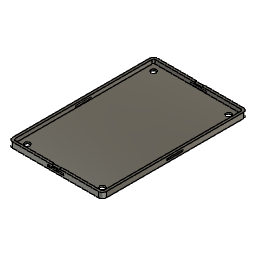
Backcover+small (Autodesk Fusion 360 design; units mm, degrees)
Autodesk Fusion 360 part; units mm, degrees
sketch "Sketch1" plane through (0, 0, 0) normal (0, 0, 1) x (1, 0, 0)
  circle A0 centre (14.5, 177.5) radius 3.5
  line L0 (7.5, 189.5) -> (118.5, 189.5)
  line L1 (123.5, 184.5) -> (123.5, 7.5)
  line L2 (118.5, 2.5) -> (7.5, 2.5)
  line L3 (2.5, 7.5) -> (2.5, 184.5)
  arc A1 (7.5, 189.5) -> (2.5, 184.5) centre (7.5, 184.5) ccw
  arc A2 (123.5, 184.5) -> (118.5, 189.5) centre (118.5, 184.5) ccw
  arc A3 (2.5, 7.5) -> (7.5, 2.5) centre (7.5, 7.5) ccw
  arc A4 (118.5, 2.5) -> (123.5, 7.5) centre (118.5, 7.5) ccw
  arc A5 (118.5, 5.5) -> (120.5, 7.5) centre (118.5, 7.5) ccw
  line L4 (120.5, 184.5) -> (120.5, 7.5)
  arc A6 (120.5, 184.5) -> (118.5, 186.5) centre (118.5, 184.5) ccw
  line L5 (7.5, 186.5) -> (118.5, 186.5)
  arc A7 (7.5, 186.5) -> (5.5, 184.5) centre (7.5, 184.5) ccw
  line L6 (5.5, 7.5) -> (5.5, 184.5)
  arc A8 (5.5, 7.5) -> (7.5, 5.5) centre (7.5, 7.5) ccw
  line L7 (118.5, 5.5) -> (7.5, 5.5)
  line L8 (63, 186.5) -> (63, 5.5)
  line L9 (5.5, 96) -> (120.5, 96)
  circle A9 centre (111.5, 177.5) radius 3.5
  circle A10 centre (14.5, 14.5) radius 3.5
  circle A11 centre (111.5, 14.5) radius 3.5
  dimension "d5" = 7
  dimension "d28" = 5
  dimension "d30" = 5
  dimension "d32" = 5
  dimension "d34" = 5
  dimension "d36" = 3
  dimension "d37" = 187
  dimension "d38" = 121
  dimension "d41" = 9
  dimension "d42" = 9
  constraint horizontal L0
  constraint perpendicular L0 L1
  constraint parallel L0 L2
  constraint parallel L1 L3
  constraint tangent L3 A1
  constraint tangent L0 A1
  constraint tangent L0 A2
  constraint tangent L1 A2
  constraint tangent L3 A3
  constraint tangent L2 A3
  constraint tangent L1 A4
  constraint tangent L2 A4
  constraint midpoint L5 L8.start
  constraint midpoint L7 L8.end
  constraint perpendicular L7 L8
  constraint midpoint L6 L9.start
  constraint midpoint L4 L9.end
  constraint perpendicular L4 L9
  constraint symmetric A0 L8 A9
  constraint symmetric A0 L9 A10
  constraint symmetric L9 A9 A11
  measures "d5" diameter of A0
  measures "d28" radius of A1
  measures "d30" radius of A2
  measures "d32" radius of A3
  measures "d34" radius of A4
  measures "d37" distance of L0 L2
  measures "d38" distance of L1 L3
  measures "d41" distance of A0.centre L5
  measures "d42" distance of A0.centre L6
extrude "Extrude5" add sketch "Sketch1" along normal blind 2 contours L0 L1 L2 L3 A1 A2 A3 A4 | A5 L4 L7 L8 L9 | L6 A8 L7 L8 L9 | L4 A6 L5 L8 L9 | L5 A7 L6 L8 L9
extrude "Extrude6" add sketch "Sketch1" along normal blind 7 contours L0 L1 L2 L3 A1 A2 A3 A4
sketch "Skizze3" plane through (2.5, 0, 0) normal (-1, 0, 0) x (0, -1, 0)
  line L0 (-184.5, 0) -> (-7.5, 0)
  line L1 (-7.5, 0) -> (-7.5, 7)
  line L2 (-7.5, 7) -> (-184.5, 7)
  line L3 (-184.5, 7) -> (-184.5, 0)
  line L4 (-184.5, 7) -> (-7.5, 0)
  line L5 (-7.5, 7) -> (-184.5, 0)
  line L6 (-85.75, 4.5) -> (-106.25, 4.5)
  line L7 (-106.25, 4.5) -> (-106.25, 2.5)
  line L8 (-106.25, 2.5) -> (-85.75, 2.5)
  line L9 (-85.75, 2.5) -> (-85.75, 4.5)
  line L10 (-85.75, 4.5) -> (-106.25, 2.5) construction
  line L11 (-106.25, 4.5) -> (-85.75, 2.5) construction
  point P0 (-96, 3.5)
  dimension "d43" = 20.5
  dimension "d44" = 2
  constraint coincident L2.end L3.start
  constraint coincident L0.end L1.start
  constraint coincident L1.end L2.start
  constraint coincident L0.start L3.end
  constraint horizontal L6
  constraint perpendicular L6 L7
  constraint parallel L6 L8
  constraint parallel L7 L9
  constraint coincident L10 P0
  constraint coincident L11 P0
  constraint midpoint L5 P0
  measures "d43" distance of L7.end L8.end
  measures "d44" distance of L6.end L7.end
extrude "Extrusion7" cut sketch "Skizze3" against normal blind 2.5 contours L4 L5 L7 | L4 L5 L7 L8 L9 | L4 L5 L9 | L4 L5 L6 L7 L9
sketch "Skizze4" plane through (0, 189.5, 0) normal (0, 1, 0) x (-1, 0, 0)
  line L0 (-118.5, 0) -> (-7.5, 0)
  line L1 (-7.5, 0) -> (-7.5, 7)
  line L2 (-7.5, 7) -> (-118.5, 7)
  line L3 (-118.5, 7) -> (-118.5, 0)
  line L4 (-118.5, 7) -> (-7.5, 0)
  line L5 (-7.5, 7) -> (-118.5, 0)
  line L6 (-52.75, 4.5) -> (-73.25, 4.5)
  line L7 (-73.25, 4.5) -> (-73.25, 2.5)
  line L8 (-73.25, 2.5) -> (-52.75, 2.5)
  line L9 (-52.75, 2.5) -> (-52.75, 4.5)
  line L10 (-52.75, 4.5) -> (-73.25, 2.5) construction
  line L11 (-73.25, 4.5) -> (-52.75, 2.5) construction
  point P0 (-63, 3.5)
  dimension "d47" = 20.5
  dimension "d48" = 2
  constraint coincident L2.end L3.start
  constraint coincident L0.end L1.start
  constraint coincident L1.end L2.start
  constraint coincident L0.start L3.end
  constraint horizontal L6
  constraint perpendicular L6 L7
  constraint parallel L6 L8
  constraint parallel L7 L9
  constraint coincident L10 P0
  constraint coincident L11 P0
  constraint midpoint L4 P0
  measures "d47" distance of L7.end L8.end
  measures "d48" distance of L6.end L7.end
extrude "Extrusion8" cut sketch "Skizze4" against normal blind 2.5 contours L4 L5 L7 | L4 L5 L7 L8 L9 | L4 L5 L9 | L4 L5 L6 L7 L9
sketch "Skizze5" plane through (0, 2.5, 0) normal (0, -1, 0) x (1, 0, 0)
  line L0 (7.5, 0) -> (118.5, 0)
  line L1 (118.5, 0) -> (118.5, 7)
  line L2 (118.5, 7) -> (7.5, 7)
  line L3 (7.5, 7) -> (7.5, 0)
  line L4 (118.5, 7) -> (7.5, 0)
  line L5 (7.5, 7) -> (118.5, 0)
  line L6 (73.25, 4.5) -> (52.75, 4.5)
  line L7 (52.75, 4.5) -> (52.75, 2.5)
  line L8 (52.75, 2.5) -> (73.25, 2.5)
  line L9 (73.25, 2.5) -> (73.25, 4.5)
  line L10 (73.25, 4.5) -> (52.75, 2.5) construction
  line L11 (52.75, 4.5) -> (73.25, 2.5) construction
  point P0 (63, 3.5)
  dimension "d51" = 20.5
  dimension "d52" = 2
  constraint coincident L1.end L2.start
  constraint coincident L0.start L3.end
  constraint coincident L2.end L3.start
  constraint coincident L0.end L1.start
  constraint horizontal L6
  constraint perpendicular L6 L7
  constraint parallel L6 L8
  constraint parallel L7 L9
  constraint coincident L10 P0
  constraint coincident L11 P0
  constraint midpoint L5 P0
  measures "d51" distance of L7.end L8.end
  measures "d52" distance of L6.end L7.end
extrude "Extrusion9" cut sketch "Skizze5" against normal blind 2.5 contours L4 L5 L7 | L4 L5 L7 L8 L9 | L4 L5 L9 | L4 L5 L6 L7 L9
sketch "Skizze6" plane through (123.5, 0, 0) normal (1, 0, 0) x (0, 1, 0)
  line L0 (7.5, 0) -> (184.5, 0)
  line L1 (184.5, 0) -> (184.5, 7)
  line L2 (184.5, 7) -> (7.5, 7)
  line L3 (7.5, 7) -> (7.5, 0)
  line L4 (7.5, 7) -> (184.5, 0)
  line L5 (184.5, 7) -> (7.5, 0)
  line L6 (106.25, 2.5) -> (85.75, 2.5)
  line L7 (85.75, 2.5) -> (85.75, 4.5)
  line L8 (85.75, 4.5) -> (106.25, 4.5)
  line L9 (106.25, 4.5) -> (106.25, 2.5)
  line L10 (106.25, 2.5) -> (85.75, 4.5) construction
  line L11 (85.75, 2.5) -> (106.25, 4.5) construction
  point P0 (96, 3.5)
  point P1 (96, 3.5)
  dimension "d55" = 20.5
  dimension "d56" = 2
  dimension "d59" = 3.5
  constraint coincident L2.end L3.start
  constraint coincident L0.end L1.start
  constraint coincident L1.end L2.start
  constraint coincident L0.start L3.end
  constraint midpoint L4 P1
  constraint horizontal L6
  constraint perpendicular L6 L7
  constraint parallel L6 L8
  constraint parallel L7 L9
  constraint coincident L10 P1
  constraint coincident L11 P1
  constraint coincident P1 P0
  measures "d55" distance of L7.end L8.end
  measures "d56" distance of L6.end L7.end
  measures "d59" distance of L0 P1
extrude "Extrusion10" cut sketch "Skizze6" against normal blind 2.5 contours L4 L5 L7 | L4 L5 L6 L7 L9 | L4 L5 L9 | L4 L5 L7 L8 L9
sketch "Cutout USB" plane through (0, 2.5, 0) normal (0, -1, 0) x (1, 0, 0)
  line L0 (52.75, 4.5) -> (73.25, 4.5)
  line L1 (73.25, 4.5) -> (73.25, 2.5)
  line L2 (73.25, 2.5) -> (52.75, 2.5)
  line L3 (52.75, 2.5) -> (52.75, 4.5)
  line L4 (7.5, 0) -> (118.5, 0)
  line L5 (118.5, 0) -> (118.5, 7)
  line L6 (118.5, 7) -> (7.5, 7)
  line L7 (7.5, 7) -> (7.5, 0)
  line L8 (58, 6.25) -> (68, 6.25)
  line L9 (68, 6.25) -> (68, 7)
  line L10 (68, 7) -> (58, 7)
  line L11 (58, 7) -> (58, 6.25)
  dimension "d64" = 10
  dimension "d65" = 0.75
  constraint horizontal L8
  constraint vertical L9
  constraint horizontal L10
  constraint vertical L11
  constraint midpoint L6 L10
  measures "d64" distance of L8.start L8.end
  measures "d65" distance of L8.start L10.end
extrude "Extrude11" cut sketch "Cutout USB" against normal blind 190 contours L6 L8 L9 L10 L11
